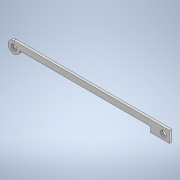
# Autodesk Inventor part: Pieza6
Saved by Autodesk Inventor 2022 (Build 260153000, 153)
## iProperties
Created: 2022-11-04
Part Number: Pieza6
Material: Genérico
Document SubType Name: Modeling
Designer: Mauricio Guerrero
Density: 1 g/cm^3
Appearance: Valor por defecto
Author: Mauricio Guerrero
## iProperties of the stored document Pieza6_3DPrint.ipt
Created: 2022-11-06
Part Number: Pieza6_3DPrint
Material: Genérico
Document SubType Name: Modeling
Designer: Mauricio Guerrero
Density: 1 g/cm^3
Appearance: Valor por defecto
Author: Mauricio Guerrero
Autodesk Inventor part; units mm, degrees
ref_plane "YZ Plane" through (0, 0, 0) normal (1, 0, 0) x (0, 1, 0)
ref_plane "XZ Plane" through (0, 0, 0) normal (0, 1, 0) x (-1, 0, 0)
ref_plane "XY Plane" through (0, 0, 0) normal (0, 0, 1) x (1, 0, 0)
sketch "Boceto1" plane through (0, 0, 0) normal (0, 0, 1) x (1, 0, 0)
  circle A0 centre (-1129.4428, 209.2327) radius 1.25
  arc A1 (-1129.4428, 211.7327) -> (-1126.9428, 209.2383) centre (-1129.4428, 209.2327) ccw
  circle A2 centre (-1065.4428, 209.2327) radius 1.25
  line L0 (-1129.4428, 211.7327) -> (-1070.7298, 211.7327)
  line L1 (-1129.1407, 209.2377) -> (-1128.1928, 209.2377)
  line L2 (-1126.9428, 209.2383) -> (-1070.9178, 209.2383)
  line L3 (-1070.9178, 209.2383) -> (-1070.9178, 206.9349)
  line L4 (-1070.9178, 206.9349) -> (-1062.8204, 206.9349)
  line L5 (-1062.8204, 206.9349) -> (-1062.8204, 211.7327)
  line L6 (-1062.8204, 211.7327) -> (-1070.7298, 211.7327)
  dimension "d9" = 5
  dimension "d10" = 2.5
  dimension "d16" = 64
  constraints: 14 end point, 3 horizontal, 3 perpendicular, 2 centre point, 2 point on circle, 1 coincident, 1 horizontal alignment, 1 tangent, 1 vertical, 3 other
  measures "d9" diameter of A1
  measures "d10" diameter of A2
  measures "d16" distance of A2.centre point (-1129.443, 209.233)
extrude "Extrusión1" add sketch "Boceto1" along normal blind 1
